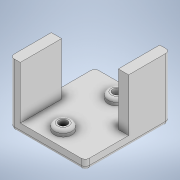
# Autodesk Inventor part: botMountThick
Saved by Autodesk Inventor 2020 (Build 240168000, 168)
## iProperties
Created: 2020-07-25
Part Number: botMountThick
Material: Generic
Document SubType Name: Modeling
Designer: PAB
Density: 1 g/cm^3
Appearance: Default
Author: PAB
Autodesk Inventor part; units mm, degrees
ref_plane "YZ Plane" through (0, 0, 0) normal (1, 0, 0) x (0, 1, 0)
ref_plane "XZ Plane" through (0, 0, 0) normal (0, 1, 0) x (-1, 0, 0)
ref_plane "XY Plane" through (0, 0, 0) normal (0, 0, 1) x (1, 0, 0)
sketch "Sketch1" plane through (0, 0, 0) normal (0, 1, 0) x (-1, 0, 0)
  line L0 (19.2, 20.5) -> (-17.2, 20.5)
  line L1 (-17.2, 20.5) -> (-17.2, -20.5)
  line L2 (-17.2, -20.5) -> (19.2, -20.5)
  line L3 (19.2, -20.5) -> (19.2, 20.5)
  point P0 (0, 0)
  dimension "d0" = 36.4
  dimension "d1" = 41
  constraints: 8 end point, 2 parallel, 1 horizontal, 1 perpendicular
  measures "d0" distance of L2.end L1.end
  measures "d1" distance of L1.end L0.end
extrude "Extrusion1" add sketch "Sketch1" along normal blind 5
sketch "Sketch2" plane through (0, 5, 0) normal (0, 1, 0) x (1, 0, 0)
  line L0 (-19.2, -20.5) -> (17.2, -20.5) projected
  line L1 (-19.2, -20.5) -> (-14.2, -20.5)
  line L2 (-14.2, -20.5) -> (-14.2, -0.5)
  line L3 (-14.2, -0.5) -> (-19.2, -0.5)
  line L4 (-19.2, -0.5) -> (-19.2, -20.5)
  line L5 (17.2, 20.5) -> (-19.2, 20.5) projected
  line L6 (17.2, 20.5) -> (12.2, 20.5)
  line L7 (12.2, 20.5) -> (12.2, 0.5)
  line L8 (12.2, 0.5) -> (17.2, 0.5)
  line L9 (17.2, 0.5) -> (17.2, 20.5)
  point P0 (0, 0)
  dimension "d4" = 5
  dimension "d5" = 20
  dimension "d6" = 5
  dimension "d7" = 20
  constraints: 16 end point, 4 parallel, 2 horizontal, 2 perpendicular
  measures "d4" distance of L3.end L2.end
  measures "d5" distance of L2.end L1.end
  measures "d6" distance of L8.end L7.end
  measures "d7" distance of L7.end L6.end
extrude "Extrusion2" add sketch "Sketch2" along normal blind 25.4
sketch "Sketch3" plane through (0, 5, 0) normal (0, 1, 0) x (1, 0, 0)
  circle A0 centre (-1, -13) radius 4.25
  circle A1 centre (-1, 13) radius 4.25
  line L0 (-14.2, -20.5) -> (-14.2, -0.5) projected
  line L1 (12.2, 20.5) -> (12.2, 0.5) projected
  point P0 (0, 0)
  dimension "d10" = 8.5
  dimension "d11" = 8.5
  dimension "d24" = 13.2
  dimension "d25" = 13.2
  constraints: 2 centre point
  measures "d10" diameter of A0
  measures "d11" diameter of A1
  measures "d24" distance from line of L0 A0.centre
  measures "d25" distance from line of L1 A1.centre
extrude "Extrusion3" add sketch "Sketch3" along normal blind 3
sketch "Sketch4" plane through (-1, 8, 13) normal (0, 1, 0) x (1, 0, 0)
  circle A0 centre (0, 0) radius 4.25 projected
  circle A1 centre (0, 0) radius 2
  circle A2 centre (0, 26) radius 4.25 projected
  circle A3 centre (0, 26) radius 2
  point P0 (1, 13)
  dimension "d14" = 4
  dimension "d15" = 4
  constraints: 2 centre point, 2 coincident
  measures "d14" diameter of A1
  measures "d15" diameter of A3
extrude "Extrusion4" cut sketch "Sketch4" against normal blind 10 contours A1 | A3
fillet "Fillet1" radius 2 8 edges at (17.2, 0, 0) (-1, 0, 20.5) (-19.2, 0, 0) (-1, 0, -20.5) (-19.2, 15.2, 20.5) (17.2, 15.2, -20.5) (-19.2, 2.5, -20.5) (17.2, 2.5, 20.5)
fillet "Fillet2" radius 1.5 2 edges at (-5.25, 8, -13) (-5.25, 8, 13)
sketch "Sketch5" plane through (0, 0, 0) normal (0, -1, 0) x (1, 0, 0)
  circle A0 centre (-1, 13) radius 2 projected
  circle A1 centre (-1, 13) radius 3
  circle A2 centre (-1, -13) radius 2 projected
  circle A3 centre (-1, -13) radius 3
  point P0 (0, 0)
  dimension "d20" = 6
  dimension "d21" = 6
  constraints: 2 centre point, 2 coincident
  measures "d20" diameter of A1
  measures "d21" diameter of A3
extrude "Extrusion5" cut sketch "Sketch5" against normal blind 3 contours A0 | A1 | A2 | A3
body "Solid1"
